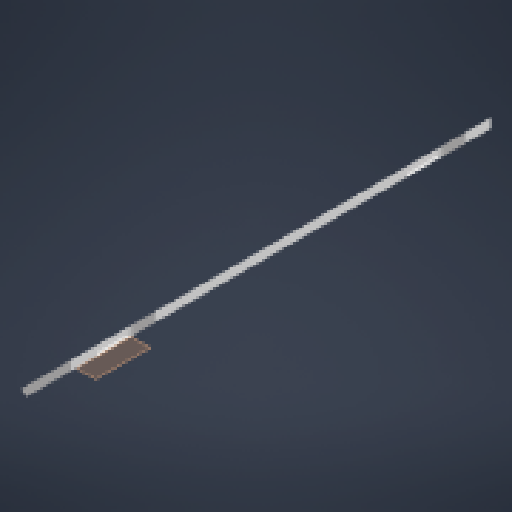
# Autodesk Inventor part: Przod
Saved by Autodesk Inventor 2023 (Build 270158000, 158)
## iProperties
Created: 2023-03-15
Part Number: Przod
Material: Generic
Document SubType Name: Modeling
Designer: Michał
Density: 1 g/cm^3
Appearance: Default
Author: Michał
Autodesk Inventor part; units mm, degrees
ref_plane "YZ Plane" through (0, 0, 0) normal (1, 0, 0) x (0, 1, 0)
ref_plane "XZ Plane" through (0, 0, 0) normal (0, 1, 0) x (-1, 0, 0)
sketch "Sketch1" plane through (0, 0, 0) normal (0, 0, 1) x (1, 0, 0)
  line L0 (7.0071, 53.5071) -> (-15, 31.5) construction
  line L1 (7, 58.5) -> (7, 55.5) construction
  line L2 (7, 57.7426) -> (-15, 35.7426)
  line L3 (-15, 35.7426) -> (-12.8787, 33.6213)
  line L4 (-12.8787, 33.6213) -> (7, 53.5)
  line L5 (7, 53.5) -> (7, 57.7426)
  line L6 (15, 58.5) -> (15, 66.5) construction
  point P0 (0, 0)
  point P1 (15, 62.5)
  dimension "d0" = 30
  dimension "d1" = 3
  constraints: 8 end point, 2 collinear, 1 midpoint, 1 parallel, 1 perpendicular
  measures "d0" horizontal distance of point (15, 62.5) L2.end
  measures "d1" distance between parallel lines of L0 L2
ref_plane "Work Plane1" through (-15, -58.5, -186) normal (0, 0, -1) x (0, 1, 0)
extrude "Extrusion1" add sketch "Sketch1" against normal up to surface (186 mm away)
ref_plane "Work Plane2" through (1.4452, 43.5974, -13.2717) normal (-0.03, 0.9995, 0) x (0.9995, 0.03, 0)
sketch "Sketch2" plane through (1.4452, 43.5974, -13.2717) normal (-0.03, 0.9995, 0) x (0.9995, 0.03, 0)
  line L0 (-4, 22) -> (-4, 0) construction
  line L1 (4, 22) -> (-4, 22) construction
  line L2 (-4, 0) -> (4, 0) construction
  line L3 (-6, 0) -> (-6, 22)
  line L4 (-4, 24) -> (5.9769, 24)
  line L5 (5.9769, 24) -> (5.9769, -2)
  line L6 (5.9769, -2) -> (-4, -2)
  line L7 (5.9769, 172.7283) -> (-16.6735, 172.7283) construction
  line L8 (-16.6735, -13.2717) -> (-16.6735, 172.7283) construction
  line L9 (5.9769, -13.2717) -> (-16.6735, -13.2717) construction
  line L10 (5.9769, -13.2717) -> (5.9769, 172.7283) construction
  arc A0 (-6, 0) -> (-4, -2) centre (-4, 0) ccw
  arc A1 (-4, 24) -> (-6, 22) centre (-4, 22) ccw
  line L11 (5.9769, 79.7283) -> (-16.6735, 79.7283)
  line L12 (-6, 159.4566) -> (-6, 137.4566)
  line L13 (-4, 135.4566) -> (5.9769, 135.4566)
  line L14 (5.9769, 135.4566) -> (5.9769, 161.4566)
  line L15 (5.9769, 161.4566) -> (-4, 161.4566)
  arc A2 (-4, 161.4566) -> (-6, 159.4566) centre (-4, 159.4566) ccw
  arc A3 (-6, 137.4566) -> (-4, 135.4566) centre (-4, 137.4566) ccw
  point P0 (-2.7531, -13.2717)
  dimension "d4" = 2
  dimension "d5" = 2
  dimension "d6" = 2
  dimension "d7" = 2
  dimension "d8" = 2
  constraints: 18 end point, 8 point on circle, 8 symmetric about line, 4 centre point, 4 tangent, 2 midpoint, 2 perpendicular, 1 collinear, 1 parallel, 2 other
  measures "d4" distance between parallel lines of L3 L0
  measures "d5" distance between parallel lines of L6 L2
  measures "d6" distance between parallel lines of L4 L1
  measures "d7" radius of A0
  measures "d8" radius of A1
extrude "Extrusion2" cut sketch "Sketch2" along normal through all
sketch "Sketch3" plane through (-15, 35.7426, -186) normal (-0.7071, 0.7071, 0) x (-0.7071, -0.7071, 0)
  circle A0 centre (-9.0711, 178) radius 2.25 projected
  circle A1 centre (-18.1127, 178) radius 2.25 projected
  circle A2 centre (-9.0711, 8) radius 2.25 projected
  circle A3 centre (-18.1127, 8) radius 2.25 projected
  point P0 (14.6673, 186)
  constraints: 4 coincident
hole "Hole1" at (-8.5858, 42.1569, -8) at (-2.1924, 48.5503, -8) at (-8.5858, 42.1569, -178) at (-2.1924, 48.5503, -178) direction (0.7071, -0.7071, 0) diameter 3.4 end through all countersink diameter 6.3 countersink angle 90 clearance for "Countersunk Flat Head Screw ISO 2009/7046" size "M3" standard "ISO"
equation "\"d5\" = d4"
equation "\"d6\" = d4"
body "Solid1"
